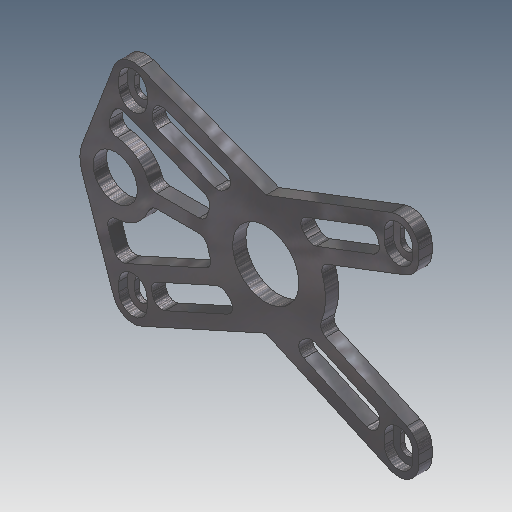
# Autodesk Inventor part: ギア支え1
Saved by Autodesk Inventor 2019.4 (Build 234330000, 330)
## iProperties
Created: 2018-08-09
Part Number: ギア支え1
Material: アルミニウム 2014-T4
Document SubType Name: Modeling
Designer: Owner
Density: 2.8 g/cm^3
Appearance: サテン
Mass: 5.01161 g
Surface Area: 45.1663 cm^2
Volume: 5.01161 cm^3
Author: Owner
Autodesk Inventor part; units mm, degrees
ref_plane "YZ Plane" through (0, 0, 0) normal (1, 0, 0) x (0, 1, 0)
ref_plane "XZ Plane" through (0, 0, 0) normal (0, 1, 0) x (-1, 0, 0)
ref_plane "XY Plane" through (0, 0, 0) normal (0, 0, 1) x (1, 0, 0)
sketch "スケッチ1" plane through (0, 0, 0) normal (0, 0, 1) x (1, 0, 0)
  circle A0 centre (0, 0) radius 5 construction
  circle A1 centre (0, 0) radius 7.5
  line L0 (-30, 20) -> (-30, 18) construction
  line L1 (-31.6, 20) -> (-31.6, 18)
  line L2 (-28.4, 18) -> (-28.4, 20)
  arc A2 (-28.4, 20) -> (-31.6, 20) centre (-30, 20) ccw
  arc A3 (-31.6, 18) -> (-28.4, 18) centre (-30, 18) ccw
  line L3 (0, 0) -> (-34, 0) construction
  line L4 (-30, -20) -> (-30, -22) construction
  line L5 (-31.6, -20) -> (-31.6, -22)
  line L6 (-28.4, -22) -> (-28.4, -20)
  arc A4 (-28.4, -20) -> (-31.6, -20) centre (-30, -20) ccw
  arc A5 (-31.6, -22) -> (-28.4, -22) centre (-30, -22) ccw
  line L7 (30, 20) -> (30, 18) construction
  line L8 (28.4, 20) -> (28.4, 18)
  line L9 (31.6, 18) -> (31.6, 20)
  arc A6 (31.6, 20) -> (28.4, 20) centre (30, 20) ccw
  arc A7 (28.4, 18) -> (31.6, 18) centre (30, 18) ccw
  line L10 (30, -20) -> (30, -22) construction
  line L11 (28.4, -20) -> (28.4, -22)
  line L12 (31.6, -22) -> (31.6, -20)
  arc A8 (31.6, -20) -> (28.4, -20) centre (30, -20) ccw
  arc A9 (28.4, -22) -> (31.6, -22) centre (30, -22) ccw
  circle A10 centre (-34, 0) radius 5
  circle A11 centre (-34, 0) radius 8
  line L13 (-25.4, 18) -> (-25.4, 20)
  arc A12 (-25.4, 20) -> (-34.6, 20) centre (-30, 20) ccw
  line L14 (-34.6, 20) -> (-34.6, 18)
  arc A13 (-34.6, 18) -> (-25.4, 18) centre (-30, 18) ccw
  line L15 (34.6, 18) -> (34.6, 20)
  arc A14 (34.6, 20) -> (25.4, 20) centre (30, 20) ccw
  line L16 (25.4, 20) -> (25.4, 18)
  arc A15 (25.4, 18) -> (34.6, 18) centre (30, 18) ccw
  line L17 (-25.4, -20) -> (-25.4, -22)
  arc A16 (-34.6, -22) -> (-25.4, -22) centre (-30, -22) ccw
  line L18 (-34.6, -22) -> (-34.6, -20)
  arc A17 (-25.4, -20) -> (-34.6, -20) centre (-30, -20) ccw
  line L19 (34.6, -22) -> (34.6, -20)
  line L20 (25.4, -20) -> (25.4, -21.6783)
  arc A18 (28.1068, -26.1924) -> (34.6, -22) centre (30, -22) ccw
  line L21 (-41.4733, 2.8547) -> (-34.2972, 21.6414)
  line L22 (-28.3632, 24.299) -> (0, 13.5)
  line L23 (0, 13.5) -> (28.3632, 24.299)
  line L24 (31.6368, 13.701) -> (11.9827, 6.218)
  line L25 (-31.6368, 13.701) -> (-11.9827, 6.218)
  line L26 (-36.4424, 7.618) -> (-33.5801, 15.1115)
  line L27 (-13.4164, 1.5) -> (-26.1419, 1.5)
  line L28 (-25.4, 19.9607) -> (-5.433, 12.3585)
  line L29 (5.433, 12.3585) -> (25.4, 19.9607)
  line L30 (-26.5388, 14.9701) -> (-10.2611, 8.7726)
  line L31 (26.5388, 14.9701) -> (10.2611, 8.7726)
  line L32 (-42, 0) -> (13.5, 0)
  line L33 (-13.4164, -1.5) -> (-26.1419, -1.5)
  line L34 (-41.5618, -2.6112) -> (-34.3481, -23.5015)
  line L35 (-36.6877, -7.535) -> (-33.4385, -16.9444)
  line L36 (-28.1068, -26.1924) -> (0, -13.5)
  line L37 (0, -13.5) -> (28.1068, -26.1924)
  line L38 (-31.8932, -15.8076) -> (-11.721, -6.6984)
  line L39 (31.8932, -15.8076) -> (11.721, -6.6984)
  line L40 (26.7279, -16.7668) -> (9.9068, -9.1708)
  line L41 (25.4, -21.6783) -> (5.0863, -12.5052)
  line L42 (-5.0863, -12.5052) -> (-25.4, -21.6783)
  line L43 (-26.7279, -16.7668) -> (-9.9068, -9.1708)
  arc A19 (-9.9068, -9.1708) -> (-5.0863, -12.5052) centre (0, 0) ccw
  arc A20 (5.0863, -12.5052) -> (9.9068, -9.1708) centre (0, 0) ccw
  arc A21 (11.721, -6.6984) -> (-11.721, -6.6984) centre (0, 0) ccw
  arc A22 (34.6, -20) -> (31.8932, -15.8076) centre (30, -20) ccw
  arc A23 (26.7279, -16.7668) -> (25.4, -20) centre (30, -20) ccw
  point P0 (-30, 19)
  point P1 (-30, -21)
  point P2 (30, 19)
  point P3 (30, -21)
  point P4 (-26, 0)
  point P5 (-39, 0)
  point P6 (-29, 0)
  point P7 (-7.5, 0)
  point P8 (7.5, 0)
  point P9 (-13.5, 0)
  dimension "d0" = 10
  dimension "d1" = 15
  dimension "d2" = 30
  dimension "d3" = 20
  dimension "d4" = 1.6
  dimension "d5" = 2
  dimension "d8" = 40
  dimension "d11" = 60
  dimension "d14" = 10
  dimension "d15" = 34
  dimension "d16" = 3
  dimension "d17" = 3
  dimension "d18" = 3
  dimension "d19" = 3
  dimension "d20" = 3
  dimension "d22" = 3
  dimension "d23" = 1.5
  dimension "d24" = 3
  dimension "d25" = 3
  dimension "d26" = 3
  dimension "d27" = 3
  dimension "d30" = 3
  dimension "d31" = 3
  dimension "d32" = 3
  dimension "d33" = 3
  dimension "d34" = 3
  dimension "d35" = 3
  dimension "d36" = 6
  constraints: 96 end point, 56 point on circle, 22 centre point, 18 tangent, 15 parallel, 13 point on line, 3 coincident, 2 concentric, 2 horizontal, 2 vertical, 2 vertical alignment, 1 collinear, 1 midpoint, 72 other
  measures "d0" diameter of A0
  measures "d1" diameter of A1
  measures "d2" horizontal distance of point (-30, 19) point (0, 0)
  measures "d3" vertical distance of point (0, 0) L0.start
  measures "d4" radius of A2
  measures "d5" distance of L0.start L0.end
  measures "d8" distance of L1.start L5.start
  measures "d11" distance of L1.start L8.start
  measures "d14" diameter of A10
  measures "d15" distance of L3.start L3.end
  measures "d17" radial gap between concentric circles of A3 A13
  measures "d18" radial gap between concentric circles of A7 A15
  measures "d19" distance between parallel lines of L6 L17
  measures "d20" radial gap between concentric circles of A9 A18
  measures "d22" distance between parallel lines of L21 L26
  measures "d23" distance between parallel lines of L3 L27
  measures "d24" distance between parallel lines of L22 L28
  measures "d25" distance between parallel lines of L25 L30
  measures "d26" distance between parallel lines of L24 L31
  measures "d27" distance between parallel lines of L23 L29
  measures "d30" distance between parallel lines of L27 L33
  measures "d31" distance between parallel lines of L34 L35
  measures "d32" distance between parallel lines of L39 L40
  measures "d33" distance between parallel lines of L37 L41
  measures "d34" distance between parallel lines of L38 L43
  measures "d35" distance between parallel lines of L36 L42
  measures "d36" radial gap between concentric circles of A1 A19
extrude "押し出し1" add sketch "スケッチ1" along normal blind 3 contours L32 A21 L39 A22 L19 A18 L37 L36 A16 L17 L42 A19 L43 A17 L38 A1 | A1 L32 A21 | A21 L33 A11 L32 | L32 A11 L27 A21 | A21 L31 A15 L24 | L32 A10 A11 | A11 L32 A10 | A15 L16 A14 L15 | L25 A13 L30 A21 | A21 L23 A14 L16 L29 | A11 L21 A12 L14 A13 L26 | L35 A17 L18 A16 L34 A11 | A13 L14 A12 L13 | A17 L17 A16 L18 | A21 L28 L13 A12 L22
fillet "フィレット1" radius 2 28 edges at (-25.4, 19.9607, 1.5) (-26.5388, 14.9701, 1.5) (-33.5801, 15.1115, 1.5) (-5.433, 12.3585, 1.5) (-10.2611, 8.7726, 1.5) (-11.9827, 6.218, 1.5) (-13.4164, 1.5, 1.5) (-13.4164, -1.5, 1.5) (-11.721, -6.6984, 1.5) (-26.1419, 1.5, 1.5) (-26.1419, -1.5, 1.5) (-36.6877, -7.535, 1.5) (-33.4385, -16.9444, 1.5) (-9.9068, -9.1708, 1.5) (-5.0863, -12.5052, 1.5) (-25.4, -21.6783, 1.5) (-26.7279, -16.7668, 1.5) (-36.4424, 7.618, 1.5) (5.0863, -12.5052, 1.5) (9.9068, -9.1708, 1.5) (26.7279, -16.7668, 1.5) (25.4, -21.6783, 1.5) (26.5388, 14.9701, 1.5) (25.4, 19.9607, 1.5) (10.2611, 8.7726, 1.5) (5.433, 12.3585, 1.5) (11.9827, 6.218, 1.5) (11.721, -6.6984, 1.5)
sketch "スケッチ2" plane through (0, 0, 3) normal (0, 0, 1) x (1, 0, 0)
  line L0 (-22.7523, 18.9526) -> (-9.1944, 13.7906) projected
  arc A0 (-8.6278, 10.3832) -> (-9.1944, 13.7906) centre (-9.906, 11.9214) ccw projected
  arc A1 (-8.6278, 10.3832) -> (-9.4066, 9.6833) centre (0, 0) ccw projected
  arc A2 (-11.5118, 9.2488) -> (-9.4066, 9.6833) centre (-10.8001, 11.1179) ccw projected
  line L1 (-11.5118, 9.2488) -> (-24.4126, 14.1606) projected
  arc A3 (-25.6098, 16.6268) -> (-24.4126, 14.1606) centre (-23.701, 16.0297) ccw projected
  arc A4 (-25.6098, 16.6268) -> (-25.4446, 17.3612) centre (-30, 18) ccw projected
  arc A5 (-22.7523, 18.9526) -> (-25.4446, 17.3612) centre (-23.4639, 17.0835) ccw projected
  line L2 (22.7176, -20.467) -> (8.6309, -14.1058) projected
  arc A6 (8.2341, -10.6981) -> (8.6309, -14.1058) centre (9.454, -12.283) ccw projected
  arc A7 (8.2341, -10.6981) -> (8.9968, -10.0651) centre (0, 0) ccw projected
  arc A8 (11.1528, -9.7335) -> (8.9968, -10.0651) centre (10.3297, -11.5563) ccw projected
  line L3 (11.1528, -9.7335) -> (24.6544, -15.8305) projected
  arc A9 (25.7006, -18.3644) -> (24.6544, -15.8305) centre (23.8313, -17.6533) ccw projected
  arc A10 (25.7006, -18.3644) -> (25.4981, -19.0551) centre (30, -20) ccw projected
  arc A11 (22.7176, -20.467) -> (25.4981, -19.0551) centre (23.5407, -18.6443) ccw projected
  arc A12 (31.6, -20) -> (28.4, -20) centre (30, -20) ccw projected
  line L4 (31.6, -20) -> (31.6, -22) projected
  arc A13 (28.4, -22) -> (31.6, -22) centre (30, -22) ccw projected
  line L5 (28.4, -22) -> (28.4, -20) projected
  arc A14 (-28.4, -20) -> (-31.6, -20) centre (-30, -20) ccw projected
  line L6 (-28.4, -20) -> (-28.4, -22) projected
  arc A15 (-31.6, -22) -> (-28.4, -22) centre (-30, -22) ccw projected
  line L7 (-31.6, -22) -> (-31.6, -20) projected
  arc A16 (31.6, 20) -> (28.4, 20) centre (30, 20) ccw projected
  line L8 (31.6, 20) -> (31.6, 18) projected
  arc A17 (28.4, 18) -> (31.6, 18) centre (30, 18) ccw projected
  line L9 (28.4, 18) -> (28.4, 20) projected
  arc A18 (-28.4, 20) -> (-31.6, 20) centre (-30, 20) ccw projected
  line L10 (-28.4, 20) -> (-28.4, 18) projected
  arc A19 (-31.6, 18) -> (-28.4, 18) centre (-30, 18) ccw projected
  line L11 (-31.6, 18) -> (-31.6, 20) projected
  line L12 (-34.2852, -14.4925) -> (-35.6124, -10.6489) projected
  arc A20 (-33.7776, -7.9969) -> (-35.6124, -10.6489) centre (-33.722, -9.9961) ccw projected
  arc A21 (-33.7776, -7.9969) -> (-26.506, -2.8) centre (-34, 0) ccw projected
  arc A22 (-24.6325, -1.5) -> (-26.506, -2.8) centre (-24.6325, -3.5) ccw projected
  line L13 (-24.6325, -1.5) -> (-15.0997, -1.5) projected
  arc A23 (-13.1513, -3.0484) -> (-15.0997, -1.5) centre (-15.0997, -3.5) ccw projected
  arc A24 (-13.1513, -3.0484) -> (-12.5482, -4.9793) centre (0, 0) ccw projected
  arc A25 (-13.5841, -7.5397) -> (-12.5482, -4.9793) centre (-14.4072, -5.7169) ccw projected
  line L14 (-13.5841, -7.5397) -> (-31.5716, -15.6624) projected
  arc A26 (-34.2852, -14.4925) -> (-31.5716, -15.6624) centre (-32.3947, -13.8397) ccw projected
  circle A27 centre (0, 0) radius 7.5 projected
  arc A28 (12.5482, -4.9793) -> (12.7514, 4.4331) centre (0, 0) ccw projected
  arc A29 (13.9288, 6.959) -> (12.7514, 4.4331) centre (14.6405, 5.0899) ccw projected
  line L15 (13.9288, 6.959) -> (31.6368, 13.701) projected
  arc A30 (31.6368, 13.701) -> (34.6, 18) centre (30, 18) ccw projected
  line L16 (34.6, 18) -> (34.6, 20) projected
  arc A31 (34.6, 20) -> (28.3632, 24.299) centre (30, 20) ccw projected
  line L17 (28.3632, 24.299) -> (0, 13.5) projected
  line L18 (0, 13.5) -> (-28.3632, 24.299) projected
  arc A32 (-28.3632, 24.299) -> (-34.2972, 21.6414) centre (-30, 20) ccw projected
  line L19 (-34.2972, 21.6414) -> (-41.4733, 2.8547) projected
  arc A33 (-41.4733, 2.8547) -> (-41.5618, -2.6112) centre (-34, 0) ccw projected
  line L20 (-41.5618, -2.6112) -> (-34.3481, -23.5015) projected
  arc A34 (-34.3481, -23.5015) -> (-28.1068, -26.1924) centre (-30, -22) ccw projected
  line L21 (-28.1068, -26.1924) -> (0, -13.5) projected
  line L22 (0, -13.5) -> (28.1068, -26.1924) projected
  arc A35 (28.1068, -26.1924) -> (34.6, -22) centre (30, -22) ccw projected
  line L23 (34.6, -22) -> (34.6, -20) projected
  arc A36 (34.6, -20) -> (31.8932, -15.8076) centre (30, -20) ccw projected
  line L24 (31.8932, -15.8076) -> (13.5841, -7.5397) projected
  arc A37 (12.5482, -4.9793) -> (13.5841, -7.5397) centre (14.4072, -5.7169) ccw projected
  arc A38 (-12.7514, 4.4331) -> (-13.1513, 3.0484) centre (0, 0) ccw projected
  arc A39 (-15.0997, 1.5) -> (-13.1513, 3.0484) centre (-15.0997, 3.5) ccw projected
  line L25 (-15.0997, 1.5) -> (-24.6325, 1.5) projected
  arc A40 (-26.506, 2.8) -> (-24.6325, 1.5) centre (-24.6325, 3.5) ccw projected
  arc A41 (-26.506, 2.8) -> (-33.5188, 7.9855) centre (-34, 0) ccw projected
  arc A42 (-35.2669, 10.6956) -> (-33.5188, 7.9855) centre (-33.3985, 9.9819) ccw projected
  line L26 (-35.2669, 10.6956) -> (-34.5138, 12.6671) projected
  arc A43 (-31.8438, 13.7857) -> (-34.5138, 12.6671) centre (-32.6455, 11.9534) ccw projected
  arc A44 (-31.8438, 13.7857) -> (-31.6368, 13.701) centre (-30, 18) ccw projected
  line L27 (-31.6368, 13.701) -> (-13.9288, 6.959) projected
  arc A45 (-12.7514, 4.4331) -> (-13.9288, 6.959) centre (-14.6405, 5.0899) ccw projected
  line L28 (9.1944, 13.7906) -> (22.7523, 18.9526) projected
  arc A46 (25.4446, 17.3612) -> (22.7523, 18.9526) centre (23.4639, 17.0835) ccw projected
  arc A47 (25.4446, 17.3612) -> (25.6098, 16.6268) centre (30, 18) ccw projected
  arc A48 (24.4126, 14.1606) -> (25.6098, 16.6268) centre (23.701, 16.0297) ccw projected
  line L29 (24.4126, 14.1606) -> (11.5118, 9.2488) projected
  arc A49 (9.4066, 9.6833) -> (11.5118, 9.2488) centre (10.8001, 11.1179) ccw projected
  arc A50 (9.4066, 9.6833) -> (8.6278, 10.3832) centre (0, 0) ccw projected
  arc A51 (9.1944, 13.7906) -> (8.6278, 10.3832) centre (9.906, 11.9214) ccw projected
  circle A52 centre (-34, 0) radius 5 projected
  line L30 (-24.6544, -15.8305) -> (-11.1528, -9.7335) projected
  arc A53 (-8.9968, -10.0651) -> (-11.1528, -9.7335) centre (-10.3297, -11.5563) ccw projected
  arc A54 (-8.9968, -10.0651) -> (-8.2341, -10.6981) centre (0, 0) ccw projected
  arc A55 (-8.6309, -14.1058) -> (-8.2341, -10.6981) centre (-9.454, -12.283) ccw projected
  line L31 (-8.6309, -14.1058) -> (-22.7176, -20.467) projected
  arc A56 (-25.4981, -19.0551) -> (-22.7176, -20.467) centre (-23.5407, -18.6443) ccw projected
  arc A57 (-25.4981, -19.0551) -> (-25.7006, -18.3644) centre (-30, -20) ccw projected
  arc A58 (-24.6544, -15.8305) -> (-25.7006, -18.3644) centre (-23.8313, -17.6533) ccw projected
  arc A59 (33.2, 20) -> (26.8, 20) centre (30, 20) ccw
  line L32 (33.2, 20) -> (33.2, 18)
  arc A60 (26.8, 18) -> (33.2, 18) centre (30, 18) ccw
  line L33 (26.8, 18) -> (26.8, 20)
  line L34 (-26.8, 18) -> (-26.8, 20)
  arc A61 (-26.8, 20) -> (-33.2, 20) centre (-30, 20) ccw
  line L35 (-33.2, 20) -> (-33.2, 18)
  arc A62 (-33.2, 18) -> (-26.8, 18) centre (-30, 18) ccw
  line L36 (-26.8, -22) -> (-26.8, -20)
  arc A63 (-26.8, -20) -> (-33.2, -20) centre (-30, -20) ccw
  line L37 (-33.2, -20) -> (-33.2, -22)
  arc A64 (-33.2, -22) -> (-26.8, -22) centre (-30, -22) ccw
  line L38 (33.2, -22) -> (33.2, -20)
  arc A65 (33.2, -20) -> (26.8, -20) centre (30, -20) ccw
  line L39 (26.8, -20) -> (26.8, -22)
  arc A66 (26.8, -22) -> (33.2, -22) centre (30, -22) ccw
  dimension "d38" = 3.2
  constraints: 16 end point, 16 point on circle, 8 centre point, 3 equal radius, 12 other
  measures "d38" radius of A59
extrude "押し出し2" cut sketch "スケッチ2" against normal blind 2 contours L32 A60 L33 A59 | A62 L35 A61 L34 | A64 L37 A63 L36 | A66 L39 A65 L38
equation "\"d8\" = 2 * d3"
equation "\"d11\" = 2 * d2"
